Autodesk Fusion 360 part; units mm, degrees
(part 2 of 2)
sketch "Sketch19" plane through (-15, 0, 0) normal (-1, 0, 0) x (0, -1, 0)
  arc A0 (60.8671, 4.9928) -> (67.6967, -30.4787) centre (60.35, -13.5) ccw
  line L0 (67.6967, -30.4787) -> (66.5054, -27.7254)
  arc A1 (60.7833, 1.9939) -> (66.5054, -27.7254) centre (60.35, -13.5) ccw
  line L1 (60.7833, 1.9939) -> (60.8671, 4.9928)
  arc A2 (64.3212, -22.6777) -> (60.6295, -3.5039) centre (60.35, -13.5) ccw
  line L2 (60.6295, -3.5039) -> (60.7833, 1.9939)
  line L3 (60.7833, 1.9939) -> (60.8671, 4.9928)
  arc A3 (60.8671, 4.9928) -> (67.6967, -30.4787) centre (60.35, -13.5) ccw
  line L4 (64.3212, -22.6777) -> (66.5054, -27.7254)
  line L5 (67.6967, -30.4787) -> (66.5054, -27.7254)
  circle A4 centre (60.35, -13.5) radius 3.925
  circle A5 centre (60.35, -13.5) radius 3.925
  point P0 (60.35, -13.5)
  constraint concentric A4 A5
extrude "Extrude17" [rolled back] along distance 3 taper angle 0
sketch "Sketch20" plane through (-18, 0, 0) normal (-1, 0, 0) x (0, -1, 0)
  arc A0 (64.3212, -22.6777) -> (60.6295, -3.5039) centre (60.35, -13.5) ccw
  line L0 (60.6295, -3.5039) -> (60.8671, 4.9928)
  arc A1 (60.8671, 4.9928) -> (67.6967, -30.4787) centre (60.35, -13.5) ccw
  line L1 (67.6967, -30.4787) -> (64.3212, -22.6777)
  circle A2 centre (60.35, -13.5) radius 3.925
  circle A3 centre (60.35, -13.5) radius 11.05
  dimension "d113" = 22.1
  constraint concentric A0 A3
  measures "d113" diameter of A3
extrude "Extrude18" [rolled back] along distance 10 taper angle 0
sketch "Sketch21" plane through (18, 0, 0) normal (1, 0, 0) x (0, 1, 0)
  line L0 (-60.8671, 4.9928) -> (-60.6295, -3.5039)
  arc A0 (-60.6295, -3.5039) -> (-64.3212, -22.6777) centre (-60.35, -13.5) ccw
  line L1 (-64.3212, -22.6777) -> (-67.6967, -30.4787)
  arc A1 (-67.6967, -30.4787) -> (-60.8671, 4.9928) centre (-60.35, -13.5) ccw
  circle A2 centre (-60.35, -13.5) radius 1
  circle A3 centre (-60.35, -13.5) radius 12.5
  dimension "d106" = 2
  dimension "d122" = 25
  constraint concentric A0 A2
  constraint concentric A2 A3
  measures "d106" diameter of A2
  measures "d122" diameter of A3
extrude "Extrude19" [rolled back] along distance -3 taper angle 0
sketch "Servo_vidacha" plane through (0, 0, -10) normal (0, 0, -1) x (1, 0, 0)
  line L0 (-19, 40.151) -> (-19, 79.85)
  line L1 (-19, 79.85) -> (-21.25, 79.85)
  line L2 (-21.25, 79.85) -> (-21.25, 86.15)
  line L3 (-21.25, 86.15) -> (-14.95, 86.15)
  arc A0 (10.3486, 85) -> (-10.3486, 85) centre (0, 67.8855) ccw
  line L4 (10.3486, 85) -> (14.95, 85)
  line L5 (14.95, 85) -> (14.95, 86.15)
  line L6 (14.95, 86.15) -> (21.25, 86.15)
  line L7 (21.25, 86.15) -> (21.25, 79.85)
  line L8 (21.25, 79.85) -> (19, 79.85)
  line L9 (19, 79.85) -> (19, 40.151)
  line L10 (19, 40.151) -> (-19, 40.151)
  circle A1 centre (0, 0) radius 31
  line L11 (23, 69.85) -> (64, 69.85)
  line L12 (64, 69.85) -> (64, 29.35)
  line L13 (64, 29.35) -> (23, 29.35)
  line L14 (23, 29.35) -> (23, 69.85)
  line L15 (23, 69.85) -> (64, 69.85)
  line L16 (64, 69.85) -> (64, 60.35)
  line L17 (64, 60.35) -> (23, 60.35)
  line L18 (23, 60.35) -> (23, 69.85)
  line L19 (18, 61.35) -> (18, 59.35)
  line L20 (19.8817, 60.35) -> (20.5, 60.35) construction
  line L21 (15, 59.35) -> (15, 61.35)
  line L22 (32.5, 77.1) -> (36.5, 77.1)
  line L23 (36.5, 77.1) -> (36.5, 22.1)
  line L24 (36.5, 22.1) -> (32.5, 22.1)
  line L25 (32.5, 22.1) -> (32.5, 77.1)
  line L26 (32.5, 22.1) -> (36.5, 29.35) construction
  line L27 (36.5, 69.85) -> (32.5, 77.1) construction
  line L28 (36.5, 77.1) -> (42, 77.1)
  line L29 (42, 77.1) -> (42, 69.85)
  line L30 (36.5, 22.1) -> (42, 22.1)
  line L31 (42, 22.1) -> (42, 29.35)
  line L32 (-14.95, 86.15) -> (-14.95, 85)
  line L33 (-14.95, 85) -> (-10.3486, 85)
  line L34 (15, 61.35) -> (18, 59.35) construction
  line L35 (18, 61.35) -> (15, 59.35) construction
  line L36 (16.5, 60.35) -> (18, 60.35) construction
  line L37 (74.8212, 51.7956) -> (74.8212, 91)
  line L38 (74.8212, 91) -> (0, 91)
  arc A2 (0, 91) -> (74.8212, 51.7956) centre (0, 0) ccw
  dimension "d109" = 41
  dimension "d110" = 40.5
  dimension "d111" = 9.5
  dimension "d112" = 5
  dimension "d125" = 27.5
  dimension "d126" = 4
  dimension "d127" = 55
  constraint horizontal L11
  constraint vertical L12
  constraint horizontal L13
  constraint vertical L14
  constraint horizontal L15
  constraint vertical L16
  constraint horizontal L17
  constraint vertical L18
  constraint coincident L12 L16.end
  constraint collinear L17 L20
  constraint horizontal L22
  constraint vertical L23
  constraint horizontal L24
  constraint vertical L25
  constraint coincident L23 L26.end
  constraint coincident L13 L26.end
  constraint coincident L15 L27.start
  constraint coincident L23 L27.start
  constraint equal L26 L27
  constraint perpendicular L23 L28
  constraint coincident L15 L29.end
  constraint perpendicular L15 L29
  constraint perpendicular L23 L30
  constraint coincident L13 L31.end
  constraint perpendicular L13 L31
  constraint coincident L21.end L34.start
  constraint coincident L19.end L34.end
  constraint coincident L19.start L35.start
  constraint coincident L21.start L35.end
  constraint midpoint L34 L36.start
  constraint midpoint L19 L36.end
  constraint collinear L17 L36
  measures "d109" distance of L11.start L11.end
  measures "d110" distance of L11.end L12.end
  measures "d111" distance of L11.end L16.end
  measures "d112" distance of L18 L19.start
  measures "d125" distance of L12 L23
  measures "d126" distance of L22.start L22.end
  measures "d127" distance of L22.end L23.end
sketch "Sketch23" plane through (-28, 0, 0) normal (-1, 0, 0) x (0, -1, 0)
  circle A0 centre (60.35, -13.5) radius 3.925
  circle A1 centre (60.35, -13.5) radius 11.15
  circle A2 centre (60.35, -13.5) radius 4.925
  circle A3 centre (60.35, -13.5) radius 3.925
  line L0 (71.5, -10) -> (71.5, -14.5264)
  line L1 (78.5, -14.5264) -> (78.5, -17.5264)
  circle A4 centre (60.35, -13.5) radius 14.15
  line L2 (78.5, -17.5264) -> (73.9151, -17.5264)
  line L3 (46.2001, -13.4416) -> (39.2001, -13.4416)
  line L4 (39.2001, -13.4416) -> (39.2001, -10.4416)
  circle A5 centre (60.35, -13.5) radius 11.5796
  line L5 (39.2001, -10.4416) -> (49.1816, -10.4416)
  line L6 (78.5, -14.5264) -> (71.884, -14.5264)
  dimension "d114" = 22.3
  dimension "d117" = 1
  dimension "d158" = 7
  dimension "d159" = 3
  dimension "d160" = 3
  dimension "d161" = 7
  dimension "d162" = 3
  constraint concentric A0 A1
  constraint concentric A1 A2
  constraint vertical L0
  constraint tangent A1 L0
  constraint concentric A1 A4
  constraint coincident A4 L2.end
  constraint perpendicular L1 L2
  constraint coincident A4 L3.start
  constraint horizontal L3
  constraint perpendicular L3 L4
  constraint vertical L1
  constraint concentric A2 A5
  constraint coincident A5 L5.end
  constraint perpendicular L4 L5
  constraint coincident A5 L6.end
  constraint perpendicular L1 L6
  measures "d114" diameter of A1
  measures "d117" distance of A2 A3
  measures "d158" distance of L0.end L1.start
  measures "d159" distance of A1 A4
  measures "d160" distance of L1.start L1.end
  measures "d161" distance of L3.start L3.end
  measures "d162" distance of L3.end L4.end
extrude "Extrude20" [rolled back] along distance -7.3 taper angle 0
extrude "Extrude21" [rolled back] along distance -10 taper angle 0
extrude "Extrude22" [rolled back] along distance -7.7 taper angle 0
extrude "Extrude23" [rolled back] along distance 8 taper angle 0
extrude "Extrude27" [rolled back] along distance 13 taper angle 0
sketch "Sketch25" plane through (0, 0, -10) normal (0, 0, -1) x (1, 0, 0)
  line L0 (-42.222, -46.1625) -> (42, -46.1625)
  line L1 (42, -46.1625) -> (42, 29.35)
  line L2 (42, 29.35) -> (-42.222, 29.35)
  line L3 (-42.222, 29.35) -> (-42.222, -46.1625)
  line L4 (-36.94, 29.35) -> (36.5, 29.35)
  line L5 (36.5, 29.35) -> (36.5, -40)
  line L6 (36.5, -40) -> (-36.94, -40)
  line L7 (-36.94, -40) -> (-36.94, 29.35)
  line L8 (64, 29.35) -> (42, 29.35)
  line L9 (42, 69.85) -> (42, 77.1)
  line L10 (36.5, 77.1) -> (36.5, 69.85)
  constraint horizontal L0
  constraint vertical L1
  constraint horizontal L2
  constraint vertical L3
  constraint horizontal L4
  constraint vertical L5
  constraint horizontal L6
  constraint vertical L7
  constraint coincident L2 L4.start
  constraint collinear L4 L8
  constraint collinear L1 L9
  constraint collinear L5 L10
extrude "Extrude28" [rolled back] along distance 17 taper angle 0
sketch "Sketch26" plane through (18, 0, 0) normal (1, 0, 0) x (0, 1, 0)
  circle A0 centre (-60.35, -13.5) radius 1
  line L0 (-60.8671, 4.9928) -> (-60.6295, -3.5039)
  arc A1 (-60.6295, -3.5039) -> (-64.3212, -22.6777) centre (-60.35, -13.5) ccw
  line L1 (-64.3212, -22.6777) -> (-67.6967, -30.4787)
  arc A2 (-67.6967, -30.4787) -> (-60.8671, 4.9928) centre (-60.35, -13.5) ccw
  circle A3 centre (-60.35, -13.5) radius 17
  line L2 (-67.35, -6.5) -> (-53.35, -6.5) construction
  line L3 (-53.35, -6.5) -> (-53.35, -20.5) construction
  line L4 (-53.35, -20.5) -> (-67.35, -20.5) construction
  line L5 (-67.35, -20.5) -> (-67.35, -6.5) construction
  line L6 (-67.35, -6.5) -> (-53.35, -20.5) construction
  line L7 (-67.35, -13.5) -> (-53.35, -13.5) construction
  line L8 (-60.35, -6.5) -> (-60.35, -20.5) construction
  circle A4 centre (-60.35, -6.5) radius 0.75
  circle A5 centre (-53.35, -13.5) radius 0.75
  circle A6 centre (-67.35, -13.5) radius 0.75
  circle A7 centre (-60.35, -20.5) radius 0.75
  dimension "d145" = 1.5
  dimension "d150" = 14
  dimension "d151" = 1.5
  dimension "d152" = 1.5
  dimension "d153" = 1.5
  dimension "d154" = 1.5
  constraint concentric A0 A3
  constraint horizontal L2
  constraint vertical L3
  constraint horizontal L4
  constraint vertical L5
  constraint midpoint A0.centre L6
  constraint midpoint L5 L7.start
  constraint midpoint L3 L7.end
  constraint midpoint L2 L8.start
  constraint midpoint L4 L8.end
  constraint coincident L8.start A4.centre
  constraint coincident L7.end A5.centre
  constraint coincident L7.start A6.centre
  constraint coincident L8.end A7.centre
  measures "d145" distance of A2 A3
  measures "d150" distance of L2.start L2.end
  measures "d151" diameter of A4
  measures "d152" diameter of A5
  measures "d153" diameter of A6
  measures "d154" diameter of A7
extrude "Extrude30" [rolled back] along distance -3 taper angle 0
extrude "Extrude34" [rolled back] along distance -7 taper angle 0
sketch "Sketch29" plane through (0, 0, -13.4416) normal (0, 0, -1) x (1, 0, 0)
  line L0 (-28, 46.2001) -> (-28, 39.2001)
  line L1 (-28, 39.2001) -> (-21, 39.2001)
  line L2 (-21, 39.2001) -> (-21, 46.2001)
  line L3 (-21, 46.2001) -> (-28, 46.2001)
  circle A0 centre (-24.5, 46.9966) radius 1.5
  dimension "d173" = 3
  measures "d173" diameter of A0
sketch "Sketch30" plane through (0, 0, -17.5264) normal (0, 0, -1) x (1, 0, 0)
  line L0 (-28, 78.5) -> (-28, 73.9151)
  line L1 (-28, 73.9151) -> (-21, 73.9151)
  line L2 (-21, 73.9151) -> (-21, 78.5)
  line L3 (-21, 78.5) -> (-28, 78.5)
  circle A0 centre (-24.5, 81.8126) radius 1.5
  dimension "d176" = 3
  measures "d176" diameter of A0
extrude "Extrude37" [rolled back] taper angle 0
sketch "Sketch31" plane through (42, 0, 0) normal (1, 0, 0) x (0, 1, 0)
  line L0 (-69.85, -10) -> (-77.1, -10)
  line L1 (-77.1, -10) -> (-77.1, -23)
  line L2 (-77.1, -23) -> (-69.85, -23)
  line L3 (-69.85, -23) -> (-69.85, -10)
  line L4 (-73.6, -2.3) -> (-25.6, -2.3) construction
  line L5 (-25.6, -2.3) -> (-25.6, -17.3) construction
  line L6 (-25.6, -17.3) -> (-73.6, -17.3) construction
  line L7 (-73.6, -17.3) -> (-73.6, -2.3) construction
  line L8 (-65.9007, -2.3) -> (-69.85, -2.3)
  circle A0 centre (-73.6, -17.3) radius 1.5
  circle A1 centre (-25.6, -17.3) radius 1.5
  dimension "d181" = 15
  dimension "d182" = 48
  dimension "d183" = 3.75
  dimension "d184" = 3
  dimension "d185" = 3
  constraint horizontal L4
  constraint vertical L5
  constraint horizontal L6
  constraint vertical L7
  constraint collinear L4 L8
  constraint coincident L6.end L7.start
  constraint coincident L5.end L6.start
  measures "d181" distance of L4.start L6.end
  measures "d182" distance of L5.end L6.end
  measures "d183" distance of L3 L7
  measures "d184" diameter of A0
  measures "d185" diameter of A1
extrude "Extrude38" [rolled back] side1offset 0 taper angle 0
extrude "Extrude39" [rolled back] along distance 23 taper angle 0
sketch "Sketch32" plane through (-23, 0, 0) normal (1, 0, 0) x (0, 1, 0)
  line L0 (-88.0454, -10) -> (-86.15, -10)
  line L1 (-86.15, -10) -> (-86.15, -5.3805)
  arc A0 (-86.15, -5.3805) -> (-88.0454, -3.3522) centre (-90.9861, -8) ccw
  line L2 (-67.9861, -2) -> (-100.9861, -2)
  line L3 (-100.9861, -2) -> (-100.9861, -16)
  line L4 (-100.9861, -16) -> (-67.9861, -16)
  line L5 (-67.9861, -16) -> (-67.9861, -2)
  line L6 (-81, -2) -> (-58.2437, -2)
  line L7 (-100.9861, -2) -> (-90.9861, -2)
  line L8 (-90.9861, -2) -> (-90.9861, -8)
  line L9 (-90.9861, -8) -> (-100.9861, -8)
  line L10 (-100.9861, -8) -> (-100.9861, -2)
  line L11 (-103, -8) -> (-66, -8)
  line L12 (-95.9861, -2) -> (-72.9861, -2)
  line L13 (-72.9861, -2) -> (-72.9861, -14.2)
  line L14 (-72.9861, -14.2) -> (-95.9861, -14.2)
  line L15 (-95.9861, -14.2) -> (-95.9861, -2)
  line L16 (-88.0454, -3.3522) -> (-88.0454, -10)
  point P0 (-90.9861, -8)
  dimension "d195" = 33
  dimension "d196" = 14
  dimension "d198" = 10
  dimension "d201" = 5
  dimension "d202" = 23
  dimension "d203" = 12.2
  constraint horizontal L2
  constraint vertical L3
  constraint horizontal L4
  constraint vertical L5
  constraint collinear L2 L6
  constraint horizontal L7
  constraint vertical L8
  constraint horizontal L9
  constraint vertical L10
  constraint collinear L9 L11
  constraint coincident P0 A0.centre
  constraint horizontal L12
  constraint vertical L13
  constraint horizontal L14
  constraint vertical L15
  constraint coincident L2 L12.start
  measures "d195" distance of L2.start L2.end
  measures "d196" distance of L2.end L3.end
  measures "d198" distance of P0 L9.end
  measures "d201" distance of L8 L15
  measures "d202" distance of L13.end L14.end
  measures "d203" distance of L12.start L14.end
extrude "Extrude40" [rolled back] along distance -35 taper angle 0
extrude "Extrude41" [rolled back] along distance -32 taper angle 0
sketch "Sketch33" plane through (0, 0, -14.2) normal (0, 0, 1) x (-1, 0, 0)
  line L0 (23, 95.9861) -> (23, 72.9861)
  line L1 (23, 72.9861) -> (55, 72.9861)
  line L2 (55, 72.9861) -> (55, 95.9861)
  line L3 (55, 95.9861) -> (23, 95.9861)
  line L4 (55, 67.8861) -> (38, 67.8861)
  line L5 (38, 67.8861) -> (38, 101.0861) construction
  line L6 (38, 101.0861) -> (55, 101.0861)
  line L7 (55, 101.0861) -> (55, 67.8861) construction
  line L8 (38, 67.8861) -> (35.4, 67.8861)
  line L9 (35.4, 67.8861) -> (35.4, 101)
  line L10 (35.4, 101) -> (38, 101)
  line L11 (38, 101) -> (38, 67.8861)
  line L12 (35.4, 67.8861) -> (26, 67.8861)
  line L13 (26, 67.8861) -> (26, 101)
  line L14 (26, 101) -> (35.4, 101)
  line L15 (35.4, 101) -> (35.4, 67.8861)
  dimension "d206" = 5.1
  dimension "d207" = 5.1
  dimension "d208" = 17
  dimension "d209" = 2.6
  constraint horizontal L4
  constraint vertical L5
  constraint horizontal L6
  constraint vertical L7
  constraint horizontal L8
  constraint vertical L9
  constraint horizontal L10
  constraint vertical L11
  constraint horizontal L12
  constraint vertical L13
  constraint horizontal L14
  constraint vertical L15
  measures "d206" distance of L1 L4
  measures "d207" distance of L3 L6
  measures "d208" distance of L4.start L4.end
  measures "d209" distance of L4.end L8.end
extrude "Extrude42" [rolled back] side1offset 0 taper angle 0
sketch "Sketch34" plane through (0, 0, -2) normal (0, 0, 1) x (-1, 0, 0)
  line L0 (35.4, 67.8861) -> (35.4, 72.9861)
  line L1 (35.4, 72.9861) -> (23, 72.9861)
  line L2 (23, 72.9861) -> (23, 88.0454)
  line L3 (58, 70.1213) -> (58, 100.9861)
  line L4 (58, 100.9861) -> (38, 100.9861)
  line L5 (38, 100.9861) -> (38, 95.9861)
  line L6 (38, 95.9861) -> (55, 95.9861)
  line L7 (55, 95.9861) -> (55, 72.9861)
  line L8 (55, 72.9861) -> (38, 72.9861)
  line L9 (38, 72.9861) -> (38, 67.8861)
  line L10 (38, 67.8861) -> (35.4, 67.8861)
  line L11 (-19, 55.451) -> (-26, 55.451)
  line L12 (-26, 55.451) -> (-26, 65.249)
  line L13 (-26, 65.249) -> (-19, 65.249)
  line L14 (-19, 65.249) -> (-19, 77.3206)
  line L15 (-19, 77.3206) -> (-15.1, 77.3206)
  line L16 (-15.1, 77.3206) -> (-15.1, 81)
  line L17 (-15.1, 81) -> (-20.1, 81)
  line L18 (-20.1, 81) -> (-20.1, 85)
  line L19 (-20.1, 85) -> (-10.3486, 85)
  arc A0 (10.3486, 85) -> (-10.3486, 85) centre (0, 67.8855) ccw
  line L20 (10.3486, 85) -> (20.1, 85)
  line L21 (20.1, 85) -> (20.1, 81)
  line L22 (20.1, 81) -> (15.1, 81)
  line L23 (15.1, 81) -> (15.1, 77.3206)
  line L24 (15.1, 77.3206) -> (19, 77.3206)
  line L25 (19, 77.3206) -> (19, 43.3794)
  line L26 (19, 43.3794) -> (-19, 43.3794)
  line L27 (-19, 43.3794) -> (-19, 55.451)
  circle A1 centre (0, 0) radius 26.55
  line L28 (35.4, 67.8861) -> (26, 67.8861)
  line L29 (26, 67.8861) -> (26, 101)
  line L30 (26, 101) -> (35.4, 101)
  line L31 (35.4, 101) -> (35.4, 67.8861)
  arc A2 (23, 88.0454) -> (0, 91) centre (0, 0) ccw
  line L32 (0, 91) -> (-74.8212, 91)
  line L33 (-74.8212, 91) -> (-74.8212, 51.7956)
  arc A3 (-74.8212, 51.7956) -> (58, 70.1213) centre (0, 0) ccw
  constraint horizontal L28
  constraint vertical L29
  constraint horizontal L30
  constraint vertical L31
  constraint coincident L0.start L10.end
extrude "Extrude43" [rolled back] along distance -8.5 taper angle 0
sketch "Sketch35" plane through (-21.25, 0, 0) normal (-1, 0, 0) x (0, -1, 0)
  line L0 (86.15, -10) -> (79.85, -10)
  line L1 (79.85, -10) -> (79.85, -42)
  line L2 (79.85, -42) -> (86.15, -42)
  line L3 (86.15, -42) -> (86.15, -10)
  line L4 (79.85, -10) -> (86.15, -10)
  line L5 (86.15, -10) -> (86.15, -42)
  line L6 (86.15, -42) -> (79.85, -42)
  line L7 (79.85, -42) -> (79.85, -10)
  constraint horizontal L4
  constraint vertical L5
  constraint horizontal L6
  constraint vertical L7
  constraint coincident L2.end L3.start
  constraint coincident L0.end L1.start
extrude "Extrude44" [rolled back] side1offset 0 taper angle 0
sketch "Sketch36" plane through (23, 0, 0) normal (-1, 0, 0) x (0, -1, 0)
  line L0 (86.15, -10) -> (91, -10)
  arc A0 (91, -2.5) -> (86.15, -5.3805) centre (90.9861, -8) ccw
  line L1 (86.15, -5.3805) -> (86.15, -10)
  line L2 (91, -10) -> (91, -2.5)
sketch "Sketch37" plane through (23, 0, 0) normal (-1, 0, 0) x (0, -1, 0)
  circle A0 centre (91, -8) radius 4.75
  dimension "d216" = 9.5
  measures "d216" diameter of A0
sketch "Sketch38" plane through (21.25, 0, 0) normal (1, 0, 0) x (0, 1, 0)
  line L0 (-79.85, -10) -> (-86.15, -10)
  line L1 (-86.15, -10) -> (-86.15, -42)
  line L2 (-86.15, -42) -> (-79.85, -42)
  line L3 (-79.85, -42) -> (-79.85, -10)
  line L4 (-81, -2) -> (-91, -2)
  line L5 (-91, -2) -> (-91, -16)
  line L6 (-91, -16) -> (-81, -16)
  line L7 (-81, -16) -> (-81, -2)
  constraint horizontal L4
  constraint vertical L5
  constraint horizontal L6
  constraint vertical L7
extrude "Extrude45" [rolled back] along distance 13 taper angle 0
extrude "Extrude46" [rolled back] along distance -9 taper angle 0
sketch "Sketch39" plane through (-20.7, 0, 0) normal (-1, 0, 0) x (0, -1, 0)
  arc A0 (63.8149, -10) -> (56.8851, -10) centre (60.35, -13.5) ccw
  line L0 (63.8149, -10) -> (70.9364, -10)
  arc A1 (70.9364, -10) -> (49.7636, -10) centre (60.35, -13.5) ccw
  line L1 (49.7636, -10) -> (56.8851, -10)
  circle A2 centre (60.35, -13.5) radius 11.05
  circle A3 centre (60.35, -13.5) radius 3.925
extrude "Extrude47" [rolled back] along distance 8 taper angle 0
sketch "Sketch40" plane through (0, 0, 0) normal (0, 0, -1) x (1, 0, 0)
  line L0 (-49.7426, 36.1401) -> (-59.9121, 50.1372)
  line L1 (-59.9121, 50.1372) -> (-56.7569, 52.4295)
  line L2 (-56.7569, 52.4295) -> (-59.8268, 56.6548)
  line L3 (-59.8268, 56.6548) -> (-63.8718, 53.7159)
  line L4 (-63.8718, 53.7159) -> (-66.223, 56.952)
  line L5 (-66.223, 56.952) -> (-58.334, 62.6837)
  arc A0 (-41.5895, 74.8492) -> (-58.334, 62.6837) centre (-39.9021, 54.9205) ccw
  line L6 (-41.5895, 74.8492) -> (-33.7005, 80.5809)
  line L7 (-33.7005, 80.5809) -> (-31.3494, 77.3449)
  line L8 (-31.3494, 77.3449) -> (-35.3944, 74.4059)
  line L9 (-35.3944, 74.4059) -> (-32.3246, 70.1806)
  line L10 (-32.3246, 70.1806) -> (-29.1694, 72.473)
  line L11 (-29.1694, 72.473) -> (-19, 58.476)
  line L12 (-19, 58.476) -> (-19, 75.7772)
  line L13 (-19, 75.7772) -> (-15.1, 75.7772)
  line L14 (-15.1, 75.7772) -> (-15.1, 81)
  line L15 (-15.1, 81) -> (-20.1, 81)
  line L16 (-20.1, 81) -> (-20.1, 85)
  line L17 (-20.1, 85) -> (-10.3486, 85)
  arc A1 (10.3486, 85) -> (-10.3486, 85) centre (0, 67.8855) ccw
  line L18 (10.3486, 85) -> (20.1, 85)
  line L19 (20.1, 85) -> (20.1, 81)
  line L20 (20.1, 81) -> (15.1, 81)
  line L21 (15.1, 81) -> (15.1, 75.7772)
  line L22 (15.1, 75.7772) -> (19, 75.7772)
  line L23 (19, 75.7772) -> (19, 58.476)
  line L24 (19, 58.476) -> (29.1694, 72.473)
  line L25 (29.1694, 72.473) -> (32.3246, 70.1806)
  line L26 (32.3246, 70.1806) -> (35.3944, 74.4059)
  line L27 (35.3944, 74.4059) -> (31.3494, 77.3449)
  line L28 (31.3494, 77.3449) -> (33.7005, 80.5809)
  line L29 (33.7005, 80.5809) -> (41.5895, 74.8492)
  arc A2 (58.334, 62.6837) -> (41.5895, 74.8492) centre (39.9021, 54.9205) ccw
  line L30 (58.334, 62.6837) -> (66.223, 56.952)
  line L31 (66.223, 56.952) -> (63.8718, 53.7159)
  line L32 (63.8718, 53.7159) -> (59.8268, 56.6548)
  line L33 (59.8268, 56.6548) -> (56.7569, 52.4295)
  line L34 (56.7569, 52.4295) -> (59.9121, 50.1372)
  line L35 (59.9121, 50.1372) -> (49.7426, 36.1401)
  line L36 (49.7426, 36.1401) -> (66.1971, 41.4865)
  line L37 (66.1971, 41.4865) -> (67.4023, 37.7774)
  line L38 (67.4023, 37.7774) -> (72.3694, 39.3913)
  line L39 (72.3694, 39.3913) -> (70.8243, 44.1466)
  line L40 (70.8243, 44.1466) -> (74.6286, 45.3827)
  line L41 (74.6286, 45.3827) -> (77.6419, 36.1086)
  arc A3 (84.0377, 16.4243) -> (77.6419, 36.1086) centre (64.563, 20.9778) ccw
  line L42 (84.0377, 16.4243) -> (87.051, 7.1502)
  line L43 (87.051, 7.1502) -> (83.2468, 5.9141)
  line L44 (83.2468, 5.9141) -> (81.7017, 10.6694)
  line L45 (81.7017, 10.6694) -> (76.7346, 9.0555)
  line L46 (76.7346, 9.0555) -> (77.9398, 5.3464)
  line L47 (77.9398, 5.3464) -> (61.4853, 0)
  line L48 (61.4853, 0) -> (77.9398, -5.3464)
  line L49 (77.9398, -5.3464) -> (76.7346, -9.0555)
  line L50 (76.7346, -9.0555) -> (81.7017, -10.6694)
  line L51 (81.7017, -10.6694) -> (83.2468, -5.9141)
  line L52 (83.2468, -5.9141) -> (87.051, -7.1502)
  line L53 (87.051, -7.1502) -> (84.0377, -16.4243)
  arc A4 (77.6419, -36.1086) -> (84.0377, -16.4243) centre (64.563, -20.9778) ccw
  line L54 (77.6419, -36.1086) -> (74.6286, -45.3827)
  line L55 (74.6286, -45.3827) -> (70.8243, -44.1466)
  line L56 (70.8243, -44.1466) -> (72.3694, -39.3913)
  line L57 (72.3694, -39.3913) -> (67.4023, -37.7774)
  line L58 (67.4023, -37.7774) -> (66.1971, -41.4865)
  line L59 (66.1971, -41.4865) -> (49.7426, -36.1401)
  line L60 (49.7426, -36.1401) -> (59.9121, -50.1372)
  line L61 (59.9121, -50.1372) -> (56.7569, -52.4295)
  line L62 (56.7569, -52.4295) -> (59.8268, -56.6548)
  line L63 (59.8268, -56.6548) -> (63.8718, -53.7159)
  line L64 (63.8718, -53.7159) -> (66.223, -56.952)
  line L65 (66.223, -56.952) -> (58.334, -62.6837)
  arc A5 (41.5895, -74.8492) -> (58.334, -62.6837) centre (39.9021, -54.9205) ccw
  line L66 (41.5895, -74.8492) -> (33.7005, -80.5809)
  line L67 (33.7005, -80.5809) -> (31.3494, -77.3449)
  line L68 (31.3494, -77.3449) -> (35.3944, -74.4059)
  line L69 (35.3944, -74.4059) -> (32.3246, -70.1806)
  line L70 (32.3246, -70.1806) -> (29.1694, -72.473)
  line L71 (29.1694, -72.473) -> (19, -58.476)
  line L72 (19, -58.476) -> (19, -75.7772)
  line L73 (19, -75.7772) -> (15.1, -75.7772)
  line L74 (15.1, -75.7772) -> (15.1, -81)
  line L75 (15.1, -81) -> (20.1, -81)
  line L76 (20.1, -81) -> (20.1, -85)
  line L77 (20.1, -85) -> (10.3486, -85)
  arc A6 (-10.3486, -85) -> (10.3486, -85) centre (0, -67.8855) ccw
  line L78 (-10.3486, -85) -> (-20.1, -85)
  line L79 (-20.1, -85) -> (-20.1, -81)
  line L80 (-20.1, -81) -> (-15.1, -81)
  line L81 (-15.1, -81) -> (-15.1, -75.7772)
  line L82 (-15.1, -75.7772) -> (-19, -75.7772)
  line L83 (-19, -75.7772) -> (-19, -58.476)
  line L84 (-19, -58.476) -> (-29.1694, -72.473)
  line L85 (-29.1694, -72.473) -> (-32.3246, -70.1806)
  line L86 (-32.3246, -70.1806) -> (-35.3944, -74.4059)
  line L87 (-35.3944, -74.4059) -> (-31.3494, -77.3449)
  line L88 (-31.3494, -77.3449) -> (-33.7005, -80.5809)
  line L89 (-33.7005, -80.5809) -> (-41.5895, -74.8492)
  arc A7 (-58.334, -62.6837) -> (-41.5895, -74.8492) centre (-39.9021, -54.9205) ccw
  line L90 (-58.334, -62.6837) -> (-66.223, -56.952)
  line L91 (-66.223, -56.952) -> (-63.8718, -53.7159)
  line L92 (-63.8718, -53.7159) -> (-59.8268, -56.6548)
  line L93 (-59.8268, -56.6548) -> (-56.7569, -52.4295)
  line L94 (-56.7569, -52.4295) -> (-59.9121, -50.1372)
  line L95 (-59.9121, -50.1372) -> (-49.7426, -36.1401)
  line L96 (-49.7426, -36.1401) -> (-66.1971, -41.4865)
  line L97 (-66.1971, -41.4865) -> (-67.4023, -37.7774)
  line L98 (-67.4023, -37.7774) -> (-72.3694, -39.3913)
  line L99 (-72.3694, -39.3913) -> (-70.8243, -44.1466)
  line L100 (-70.8243, -44.1466) -> (-74.6286, -45.3827)
  line L101 (-74.6286, -45.3827) -> (-77.6419, -36.1086)
  arc A8 (-84.0377, -16.4243) -> (-77.6419, -36.1086) centre (-64.563, -20.9778) ccw
  line L102 (-84.0377, -16.4243) -> (-87.051, -7.1502)
  line L103 (-87.051, -7.1502) -> (-83.2468, -5.9141)
  line L104 (-83.2468, -5.9141) -> (-81.7017, -10.6694)
  line L105 (-81.7017, -10.6694) -> (-76.7346, -9.0555)
  line L106 (-76.7346, -9.0555) -> (-77.9398, -5.3464)
  line L107 (-77.9398, -5.3464) -> (-61.4853, 0)
  line L108 (-61.4853, 0) -> (-77.9398, 5.3464)
  line L109 (-77.9398, 5.3464) -> (-76.7346, 9.0555)
  line L110 (-76.7346, 9.0555) -> (-81.7017, 10.6694)
  line L111 (-81.7017, 10.6694) -> (-83.2468, 5.9141)
  line L112 (-83.2468, 5.9141) -> (-87.051, 7.1502)
  line L113 (-87.051, 7.1502) -> (-84.0377, 16.4243)
  arc A9 (-77.6419, 36.1086) -> (-84.0377, 16.4243) centre (-64.563, 20.9778) ccw
  line L114 (-77.6419, 36.1086) -> (-74.6286, 45.3827)
  line L115 (-74.6286, 45.3827) -> (-70.8243, 44.1466)
  line L116 (-70.8243, 44.1466) -> (-72.3694, 39.3913)
  line L117 (-72.3694, 39.3913) -> (-67.4023, 37.7774)
  line L118 (-67.4023, 37.7774) -> (-66.1971, 41.4865)
  line L119 (-66.1971, 41.4865) -> (-49.7426, 36.1401)
  circle A10 centre (0, 0) radius 91
  line L120 (0, 0) -> (0, -110) construction
  line L121 (-3, -97.9505) -> (3, -97.9505)
  line L122 (3, -97.9505) -> (3, -90.9505)
  line L123 (3, -90.9505) -> (-3, -90.9505)
  line L124 (-3, -90.9505) -> (-3, -97.9505)
  dimension "d223" = 7
  dimension "d224" = 6
  dimension "d225" = 3
  constraint coincident A10.centre L120.start
  constraint vertical L120
  constraint horizontal L121
  constraint vertical L122
  constraint horizontal L123
  constraint vertical L124
  constraint coincident A10 L122.end
  measures "d223" distance of L121.end L122.end
  measures "d224" distance of L121.start L121.end
  measures "d225" distance of L120 L122
extrude "Extrude48" [rolled back] along distance -3.5 taper angle 0
fillet "Fillet2" [rolled back] radius 1.5
pattern_circular "C-Pattern3" [rolled back] count u 10 total angle 360
sketch "Sketch41" plane through (0, 0, -10) normal (0, 0, -1) x (1, 0, 0)
  circle A0 centre (0, 0) radius 31
  line L0 (-19, 62.1264) -> (-28.7, 62.1264)
  line L1 (-28.7, 62.1264) -> (-28.7, 67.8861)
  line L2 (-28.7, 67.8861) -> (-38, 67.8861)
  line L3 (-38, 67.8861) -> (-38, 67.9861)
  line L4 (-38, 67.9861) -> (-58, 67.9861)
  line L5 (-58, 67.9861) -> (-58, 70.1213)
  line L6 (64, 69.85) -> (64, 29.35)
  line L7 (64, 29.35) -> (42, 29.35)
  line L8 (42, 29.35) -> (42, -46.1625)
  line L9 (42, -46.1625) -> (-42.222, -46.1625)
  line L10 (-42.222, -46.1625) -> (-42.222, 29.35)
  line L11 (-42.222, 29.35) -> (-36.94, 29.35)
  line L12 (-36.94, 29.35) -> (-36.94, -40)
  line L13 (-36.94, -40) -> (36.5, -40)
  line L14 (36.5, -40) -> (36.5, 22.1)
  line L15 (36.5, 22.1) -> (32.5, 22.1)
  line L16 (32.5, 22.1) -> (32.5, 29.35)
  line L17 (32.5, 29.35) -> (23, 29.35)
  line L18 (23, 29.35) -> (23, 48.35)
  line L19 (19, 72.35) -> (26, 72.35)
  line L20 (19, 79.85) -> (19, 72.35)
  line L21 (19, 40.151) -> (-19, 40.151)
  line L22 (-19, 40.151) -> (-19, 56.8851)
  line L23 (-19, 56.8851) -> (-20.7, 56.8851)
  line L24 (-20.7, 56.8851) -> (-20.7, 49.7636)
  line L25 (-20.7, 49.7636) -> (-28, 49.7636)
  line L26 (-28, 49.7636) -> (-28, 49.8689)
  line L27 (-28, 49.8689) -> (-28.7, 49.8689)
  line L28 (-28.7, 49.8689) -> (-28.7, 58.5736)
  line L29 (-28.7, 58.5736) -> (-19, 58.5736)
  line L30 (-19, 58.5736) -> (-19, 62.1264)
  line L31 (54.6947, -72.7289) -> (58.7874, -78.362)
  line L32 (56.3604, -80.1253) -> (52.2677, -74.4922)
  line L33 (56.3604, -80.1253) -> (50.0179, -71.3957)
  line L34 (54.6947, -72.7289) -> (52.4778, -69.6775)
  line L35 (52.4778, -69.6775) -> (50.0179, -71.3957)
  arc A1 (-58, 70.1213) -> (74.8212, 51.7956) centre (0, 0) ccw
  line L36 (74.8212, 51.7956) -> (74.8212, 91)
  line L37 (74.8212, 91) -> (34.25, 91)
  line L38 (34.25, 91) -> (34.25, 81)
  line L39 (34.25, 81) -> (21.25, 81)
  line L40 (21.25, 81) -> (21.25, 79.85)
  line L41 (21.25, 79.85) -> (19, 79.85)
  line L42 (26, 72.35) -> (26, 69.85)
  line L43 (26, 69.85) -> (32.5, 69.85)
  line L44 (32.5, 69.85) -> (32.5, 77.1)
  line L45 (32.5, 77.1) -> (36.5, 77.1)
  line L46 (36.5, 77.1) -> (42, 77.1)
  line L47 (42, 77.1) -> (42, 69.85)
  line L48 (42, 69.85) -> (64, 69.85)
  line L49 (23, 48.35) -> (19, 48.35)
  line L50 (19, 48.35) -> (19, 40.151)
  constraint coincident L32.start L33.start
  constraint parallel L32 L33
  constraint coincident L31.start L34.start
  constraint parallel L31 L34
extrude "Extrude49" [rolled back] along distance -1 taper angle 0
sketch "Sketch42" plane through (0, 0, 8) normal (0, 0, 1) x (-1, 0, 0)
  arc A0 (-41.5895, 74.8492) -> (-58.334, 62.6837) centre (-39.9021, 54.9205) ccw
  line L0 (-41.5895, 74.8492) -> (-37.8669, 77.5538)
  line L1 (-37.8669, 77.5538) -> (-38.5429, 78.4842)
  line L2 (-38.5429, 78.4842) -> (-33.4461, 82.1873)
  line L3 (-33.4461, 82.1873) -> (-29.743, 77.0904)
  arc A1 (-21.25, 79.85) -> (-29.743, 77.0904) centre (-19.1862, 59.0492) ccw
  line L4 (-21.25, 79.85) -> (-21.25, 86.15)
  line L5 (-21.25, 86.15) -> (-14.95, 86.15)
  line L6 (-14.95, 86.15) -> (-14.95, 85)
  line L7 (-14.95, 85) -> (-10.3486, 85)
  arc A2 (10.3486, 85) -> (-10.3486, 85) centre (0, 67.8855) ccw
  line L8 (10.3486, 85) -> (14.95, 85)
  line L9 (14.95, 85) -> (14.95, 86.15)
  line L10 (14.95, 86.15) -> (21.25, 86.15)
  line L11 (21.25, 86.15) -> (21.25, 79.85)
  arc A3 (29.743, 77.0904) -> (21.25, 79.85) centre (19.1862, 59.0492) ccw
  line L12 (29.743, 77.0904) -> (33.4461, 82.1873)
  line L13 (33.4461, 82.1873) -> (38.5429, 78.4842)
  line L14 (38.5429, 78.4842) -> (37.8669, 77.5538)
  line L15 (37.8669, 77.5538) -> (41.5895, 74.8492)
  arc A4 (58.334, 62.6837) -> (41.5895, 74.8492) centre (39.9021, 54.9205) ccw
  line L16 (58.334, 62.6837) -> (62.0566, 59.9791)
  line L17 (62.0566, 59.9791) -> (62.7325, 60.9094)
  line L18 (62.7325, 60.9094) -> (67.8293, 57.2064)
  line L19 (67.8293, 57.2064) -> (64.1263, 52.1096)
  arc A5 (69.3753, 44.885) -> (64.1263, 52.1096) centre (50.2302, 36.4944) ccw
  line L20 (69.3753, 44.885) -> (75.3669, 46.8318)
  line L21 (75.3669, 46.8318) -> (77.3137, 40.8401)
  line L22 (77.3137, 40.8401) -> (76.22, 40.4847)
  line L23 (76.22, 40.4847) -> (77.6419, 36.1086)
  arc A6 (84.0377, 16.4243) -> (77.6419, 36.1086) centre (64.563, 20.9778) ccw
  line L24 (84.0377, 16.4243) -> (85.4596, 12.0481)
  line L25 (85.4596, 12.0481) -> (86.5533, 12.4035)
  line L26 (86.5533, 12.4035) -> (88.5001, 6.4119)
  line L27 (88.5001, 6.4119) -> (82.5085, 4.4651)
  arc A7 (82.5085, -4.4651) -> (82.5085, 4.4651) centre (62.088, 0) ccw
  line L28 (82.5085, -4.4651) -> (88.5001, -6.4119)
  line L29 (88.5001, -6.4119) -> (86.5533, -12.4035)
  line L30 (86.5533, -12.4035) -> (85.4596, -12.0481)
  line L31 (85.4596, -12.0481) -> (84.0377, -16.4243)
  arc A8 (77.6419, -36.1086) -> (84.0377, -16.4243) centre (64.563, -20.9778) ccw
  line L32 (77.6419, -36.1086) -> (76.22, -40.4847)
  line L33 (76.22, -40.4847) -> (77.3137, -40.8401)
  line L34 (77.3137, -40.8401) -> (75.3669, -46.8318)
  line L35 (75.3669, -46.8318) -> (69.3753, -44.885)
  arc A9 (64.1263, -52.1096) -> (69.3753, -44.885) centre (50.2302, -36.4944) ccw
  line L36 (64.1263, -52.1096) -> (67.8293, -57.2064)
  line L37 (67.8293, -57.2064) -> (62.7325, -60.9094)
  line L38 (62.7325, -60.9094) -> (62.0566, -59.9791)
  line L39 (62.0566, -59.9791) -> (58.334, -62.6837)
  arc A10 (41.5895, -74.8492) -> (58.334, -62.6837) centre (39.9021, -54.9205) ccw
  line L40 (41.5895, -74.8492) -> (37.8669, -77.5538)
  line L41 (37.8669, -77.5538) -> (38.5429, -78.4842)
  line L42 (38.5429, -78.4842) -> (33.4461, -82.1873)
  line L43 (33.4461, -82.1873) -> (29.743, -77.0904)
  arc A11 (21.25, -79.85) -> (29.743, -77.0904) centre (19.1862, -59.0492) ccw
  line L44 (21.25, -79.85) -> (21.25, -86.15)
  line L45 (21.25, -86.15) -> (14.95, -86.15)
  line L46 (14.95, -86.15) -> (14.95, -85)
  line L47 (14.95, -85) -> (10.3486, -85)
  arc A12 (-10.3486, -85) -> (10.3486, -85) centre (0, -67.8855) ccw
  line L48 (-10.3486, -85) -> (-14.95, -85)
  line L49 (-14.95, -85) -> (-14.95, -86.15)
  line L50 (-14.95, -86.15) -> (-21.25, -86.15)
  line L51 (-21.25, -86.15) -> (-21.25, -79.85)
  arc A13 (-29.743, -77.0904) -> (-21.25, -79.85) centre (-19.1862, -59.0492) ccw
  line L52 (-29.743, -77.0904) -> (-33.4461, -82.1873)
  line L53 (-33.4461, -82.1873) -> (-38.5429, -78.4842)
  line L54 (-38.5429, -78.4842) -> (-37.8669, -77.5538)
  line L55 (-37.8669, -77.5538) -> (-41.5895, -74.8492)
  arc A14 (-58.334, -62.6837) -> (-41.5895, -74.8492) centre (-39.9021, -54.9205) ccw
  line L56 (-58.334, -62.6837) -> (-62.0566, -59.9791)
  line L57 (-62.0566, -59.9791) -> (-62.7325, -60.9094)
  line L58 (-62.7325, -60.9094) -> (-67.8293, -57.2064)
  line L59 (-67.8293, -57.2064) -> (-64.1263, -52.1096)
  arc A15 (-69.3753, -44.885) -> (-64.1263, -52.1096) centre (-50.2302, -36.4944) ccw
  line L60 (-69.3753, -44.885) -> (-75.3669, -46.8318)
  line L61 (-75.3669, -46.8318) -> (-77.3137, -40.8401)
  line L62 (-77.3137, -40.8401) -> (-76.22, -40.4847)
  line L63 (-76.22, -40.4847) -> (-77.6419, -36.1086)
  arc A16 (-84.0377, -16.4243) -> (-77.6419, -36.1086) centre (-64.563, -20.9778) ccw
  line L64 (-84.0377, -16.4243) -> (-85.4596, -12.0481)
  line L65 (-85.4596, -12.0481) -> (-86.5533, -12.4035)
  line L66 (-86.5533, -12.4035) -> (-88.5001, -6.4119)
  line L67 (-88.5001, -6.4119) -> (-82.5085, -4.4651)
  arc A17 (-82.5085, 4.4651) -> (-82.5085, -4.4651) centre (-62.088, 0) ccw
  line L68 (-82.5085, 4.4651) -> (-88.5001, 6.4119)
  line L69 (-88.5001, 6.4119) -> (-86.5533, 12.4035)
  line L70 (-86.5533, 12.4035) -> (-85.4596, 12.0481)
  line L71 (-85.4596, 12.0481) -> (-84.0377, 16.4243)
  arc A18 (-77.6419, 36.1086) -> (-84.0377, 16.4243) centre (-64.563, 20.9778) ccw
  line L72 (-77.6419, 36.1086) -> (-76.22, 40.4847)
  line L73 (-76.22, 40.4847) -> (-77.3137, 40.8401)
  line L74 (-77.3137, 40.8401) -> (-75.3669, 46.8318)
  line L75 (-75.3669, 46.8318) -> (-69.3753, 44.885)
  arc A19 (-64.1263, 52.1096) -> (-69.3753, 44.885) centre (-50.2302, 36.4944) ccw
  line L76 (-64.1263, 52.1096) -> (-67.8293, 57.2064)
  line L77 (-67.8293, 57.2064) -> (-62.7325, 60.9094)
  line L78 (-62.7325, 60.9094) -> (-62.0566, 59.9791)
  line L79 (-62.0566, 59.9791) -> (-58.334, 62.6837)
  circle A20 centre (0, 0) radius 91
  line L80 (-59.1508, -55.7244) -> (-64.1263, -52.1096)
  line L81 (-64.1263, -52.1096) -> (-67.8293, -57.2064)
  line L82 (-67.8293, -57.2064) -> (-62.7325, -60.9094)
  line L83 (-62.7325, -60.9094) -> (-62.0566, -59.9791)
  line L84 (-62.0566, -59.9791) -> (-66.223, -56.952)
  line L85 (-66.223, -56.952) -> (-63.8718, -53.7159)
  line L86 (-63.8718, -53.7159) -> (-59.8268, -56.6548)
  line L87 (-59.8268, -56.6548) -> (-59.1508, -55.7244)
  line L88 (-62.0566, -59.9791) -> (-60.843, -60.8607)
  line L89 (-60.843, -60.8607) -> (-62.4007, -63.0046)
  line L90 (-62.4007, -63.0046) -> (-69.9245, -57.5382)
  line L91 (-69.9245, -57.5382) -> (-64.4581, -50.0144)
  line L92 (-64.4581, -50.0144) -> (-58.2822, -54.5015)
  line L93 (-58.2822, -54.5015) -> (-59.1508, -55.7244)
  line L94 (-35.3944, -74.4059) -> (-31.3494, -77.3449)
  line L95 (-31.3494, -77.3449) -> (-33.7005, -80.5809)
  line L96 (-33.7005, -80.5809) -> (-37.8669, -77.5538)
  line L97 (-37.8669, -77.5538) -> (-38.5429, -78.4842)
  line L98 (-38.5429, -78.4842) -> (-33.4461, -82.1873)
  line L99 (-33.4461, -82.1873) -> (-29.743, -77.0904)
  line L100 (-29.743, -77.0904) -> (-34.7185, -73.4756)
  line L101 (-34.7185, -73.4756) -> (-35.3944, -74.4059)
  line L102 (-34.7185, -73.4756) -> (-33.8368, -72.262)
  line L103 (-33.8368, -72.262) -> (-27.6478, -76.7586)
  line L104 (-27.6478, -76.7586) -> (-33.1142, -84.2825)
  line L105 (-33.1142, -84.2825) -> (-40.6381, -78.8161)
  line L106 (-40.6381, -78.8161) -> (-39.0805, -76.6722)
  line L107 (-37.8669, -77.5538) -> (-39.0805, -76.6722)
  dimension "d236" = 1.5
  dimension "d237" = 1.5
  dimension "d238" = 1.5
  dimension "d239" = 1.5
  dimension "d240" = 1.5
  dimension "d241" = 1.5
  dimension "d242" = 1.5
  dimension "d243" = 1.5
  constraint coincident L56.end L57.start
  constraint coincident L56 L88.end
  constraint perpendicular L83 L88
  constraint perpendicular L56 L89
  constraint perpendicular L89 L90
  constraint perpendicular L56 L91
  constraint perpendicular L89 L92
  constraint coincident L80.start L87.end
  constraint coincident L100.end L101.start
  constraint perpendicular L100 L102
  constraint perpendicular L102 L103
  constraint perpendicular L103 L104
  constraint perpendicular L104 L105
  constraint coincident L55 L106.end
  constraint perpendicular L55 L106
  constraint coincident L54.end L55.start
  measures "d236" distance of L82 L90
  measures "d237" distance of L81 L91
  measures "d238" distance of L80 L92
  measures "d239" distance of L56.end L89
  measures "d240" distance of L98 L105
  measures "d241" distance of L106 L54.end
  measures "d242" distance of L100 L103
  measures "d243" distance of L99 L104
extrude "Extrude50" [rolled back] along distance 3 taper angle 0
pattern_circular "C-Pattern4" [rolled back] count u 10 total angle 360
hidden bodies 1
equation "d3 = ( 37.2 / 2 ) * 1 mm"
equation "d140 = 32 mm - 15 mm"
named bodies: "Капсула 1", "Нижняя турель капсул", "Основа приема капсул", "Капсула 2"
